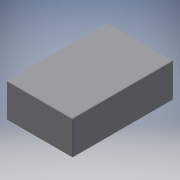
# Autodesk Inventor part: Waterproof box
Saved by Autodesk Inventor 2018 (Build 220112000, 112)
## iProperties
Created: 2018-08-07
Part Number: Waterproof box
Material: Generic
Document SubType Name: Modeling
Designer: ruben
Density: 1 g/cm^3
Sheet Metal Rule: Default_mm
Appearance: Default
Author: ruben
Autodesk Inventor part; units mm, degrees
ref_plane "YZ Plane" through (0, 0, 0) normal (1, 0, 0) x (0, 1, 0)
ref_plane "XZ Plane" through (0, 0, 0) normal (0, 1, 0) x (-1, 0, 0)
ref_plane "XY Plane" through (0, 0, 0) normal (0, 0, 1) x (1, 0, 0)
sketch "Sketch3" plane through (0, 0, 0) normal (0, 0, 1) x (1, 0, 0)
  line L0 (0, -102.2) -> (0, 102.2) projected
  line L1 (-155.4, 0) -> (155.4, 0) projected
  line L2 (-111, 73) -> (111, 73)
  line L3 (111, 73) -> (111, -73)
  line L4 (111, -73) -> (-111, -73)
  line L5 (-111, -73) -> (-111, 73)
  line L6 (-111, 73) -> (111, -73) construction
  line L7 (111, 73) -> (-111, -73) construction
  point P0 (0, 0)
  dimension "d0" = 222
  dimension "d1" = 146
  constraints: 12 end point, 2 midpoint, 2 parallel, 1 horizontal, 1 perpendicular
  measures "d0" distance of L3.end L4.end
  measures "d1" distance of L2.end L3.end
extrude "Extrusion1" add sketch "Sketch3" along normal blind 75
fillet "Fillet1" radius 2 12 edges at (-111, 73, 37.5) (0, 73, 75) (-111, 0, 75) (0, 73, 0) (-111, 0, 0) (-111, -73, 37.5) (0, -73, 0) (0, -73, 75) (111, 73, 37.5) (111, 0, 75) (111, 0, 0) (111, -73, 37.5)
equation "\"BendRadius\" = Thickness"
equation "\"BendReliefWidth\" = Thickness"
equation "\"BendReliefDepth\" = 0.5 * Thickness"
equation "\"CornerReliefSize\" = 4 * Thickness"
equation "\"MinimumRemnant\" = 2 * Thickness"
equation "\"TransitionRadius\" = BendRadius"
equation "\"JacobiRadiusSize\" = BendRadius"
equation "\"GapSize\" = Thickness"
equation "\"Thickness\" = 0.5"
body "Solid1"
